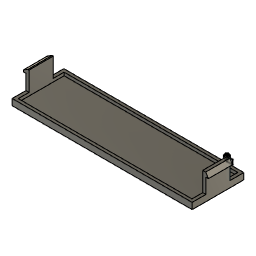
cover-5.25 (Autodesk Fusion 360 design; units mm, degrees)
Autodesk Fusion 360 part; units mm, degrees
sketch "Base" plane through (0, 0, 0) normal (0, 0, 1) x (1, 0, 0)
  line L0 (1.7267, 45) -> (150.7267, 45)
  line L1 (150.7267, 45) -> (150.7267, 2.25)
  line L2 (150.7267, 2.25) -> (1.7267, 2.25)
  line L3 (1.7267, 2.25) -> (1.7267, 45)
  dimension "d1" = 149
  dimension "d2" = 42.75
  constraint horizontal L0
  constraint vertical L1
  constraint horizontal L2
  constraint vertical L3
  measures "d1" distance of L1 L3
  measures "d2" distance of L0 L2
extrude "Extrude1" add sketch "Base" along normal blind 5.2
sketch "Frame" plane through (0, 0, 5.2) normal (0, 0, 1) x (-1, 0, 0)
  line L0 (-1.7267, -2.25) -> (-150.7267, -2.25)
  line L1 (-150.7267, -2.25) -> (-150.7267, -45)
  line L2 (-150.7267, -45) -> (-1.7267, -45)
  line L3 (-1.7267, -45) -> (-1.7267, -2.25)
  line L4 (-4.3267, -42.6) -> (-148.1267, -42.6)
  line L5 (-148.1267, -42.6) -> (-148.1267, -4.65)
  line L6 (-148.1267, -4.65) -> (-4.3267, -4.65)
  line L7 (-4.3267, -4.65) -> (-4.3267, -42.6)
  dimension "d5" = 2.4
  dimension "d6" = 2.6
  dimension "d7" = 2.4
  dimension "d8" = 2.6
  constraint horizontal L4
  constraint vertical L5
  constraint horizontal L6
  constraint vertical L7
  measures "d5" distance of L2 L4
  measures "d6" distance of L3 L7
  measures "d7" distance of L0 L6
  measures "d8" distance of L1 L5
extrude "Extrude2" cut sketch "Frame" against normal blind 2.6 contours L4 L5 L6 L7
sketch "Hook" plane through (0, 0, 5.2) normal (0, 0, 1) x (-1, 0, 0)
  line L0 (-148.1267, -42.6) -> (-148.1267, -4.65)
  line L1 (-148.1267, -4.65) -> (-4.3267, -4.65)
  line L2 (-4.3267, -4.65) -> (-4.3267, -42.6)
  line L3 (-4.3267, -42.6) -> (-148.1267, -42.6)
  line L4 (-1.7267, -2.25) -> (-150.7267, -2.25)
  line L5 (-150.7267, -2.25) -> (-150.7267, -45)
  line L6 (-150.7267, -45) -> (-1.7267, -45)
  line L7 (-1.7267, -45) -> (-1.7267, -2.25)
  line L8 (-1.7267, -33.625) -> (-4.3267, -33.625)
  line L9 (-4.3267, -13.625) -> (-1.7267, -13.625)
  line L10 (-148.1267, -33.625) -> (-150.7267, -33.625)
  line L11 (-148.1267, -13.625) -> (-150.7267, -13.625)
  dimension "d11" = 20
  dimension "d12" = 11.375
  dimension "d13" = 12.2767
  dimension "d14" = 11.375
  dimension "d15" = 20
  constraint coincident L7 L8.start
  constraint coincident L2 L8.end
  constraint perpendicular L2 L8
  constraint coincident L2 L9.start
  constraint coincident L7 L9.end
  constraint perpendicular L7 L9
  constraint coincident L5 L10.end
  constraint perpendicular L5 L10
  constraint coincident L0 L11.start
  constraint coincident L5 L11.end
  constraint perpendicular L5 L11
  measures "d11" distance of L8 L9
  measures "d12" distance of L6 L8
  measures "d14" distance of L6 L10.end
  measures "d15" distance of L10 L11
extrude "Extrude3" add sketch "Hook" along normal blind 16 contours L0 L5 L10 L11 | L2 L7 L8 L9
sketch "Hook Left" plane through (0, 33.625, 0) normal (0, 1, 0) x (-1, 0, 0)
  line L0 (-150.7267, 5.2) -> (-148.1267, 5.2)
  line L1 (-148.1267, 5.2) -> (-148.1267, 21.2)
  line L2 (-148.1267, 21.2) -> (-150.7267, 21.2)
  line L3 (-150.7267, 21.2) -> (-150.7267, 5.2)
  line L4 (-148.1267, 21.2) -> (-152.7767, 21.2)
  line L5 (-152.7767, 21.2) -> (-152.7767, 17.55)
  line L6 (-152.7767, 17.55) -> (-148.1267, 17.55)
  line L7 (-148.1267, 17.55) -> (-148.1267, 21.2)
  dimension "d18" = 3.65
  dimension "d19" = 4.65
  constraint horizontal L4
  constraint vertical L5
  constraint horizontal L6
  constraint vertical L7
  constraint coincident L1.end L2.start
  measures "d18" distance of L1.end L6.end
  measures "d19" distance of L5 L7
extrude "Extrude4" add sketch "Hook Left" against normal blind 20 contours L3 L4 L5 L6
sketch "Hook Right" plane through (0, 33.625, 0) normal (0, 1, 0) x (-1, 0, 0)
  line L0 (-4.3267, 5.2) -> (-1.7267, 5.2)
  line L1 (-1.7267, 5.2) -> (-1.7267, 21.2)
  line L2 (-1.7267, 21.2) -> (-4.3267, 21.2)
  line L3 (-4.3267, 21.2) -> (-4.3267, 5.2)
  line L4 (-4.3267, 21.2) -> (0.3233, 21.2)
  line L5 (0.3233, 21.2) -> (0.3233, 17.55)
  line L6 (0.3233, 17.55) -> (-4.3267, 17.55)
  line L7 (-4.3267, 17.55) -> (-4.3267, 21.2)
  dimension "d22" = 3.65
  dimension "d23" = 4.65
  constraint horizontal L4
  constraint vertical L5
  constraint horizontal L6
  constraint vertical L7
  constraint coincident L2.end L3.start
  measures "d22" distance of L2.end L6.end
  measures "d23" distance of L2.end L4.end
extrude "Extrude5" add sketch "Hook Right" against normal blind 20 contours L1 L4 L5 L6
chamfer "Chamfer1" distance 3.65 distance2 2.2 2 edges at (152.7767, 23.625, 21.2) (-0.3233, 23.625, 21.2) measured on face at (152.7767, 26.9583, 19.9833) measured on face at (2.7767, 20.2917, 21.2)
named bodies: "5.25 Cover"
